Autodesk Inventor part; units mm, degrees
(part 8 of 8)
  spline S282 degree 3 poles (-4.5229, -9.4251) (-4.5278, -9.4188) (-4.5373, -9.4067) (-4.5516, -9.3896) (-4.5651, -9.3741) (-4.5784, -9.3606) (-4.5908, -9.3484) (-4.6028, -9.3379) (-4.6143, -9.3292) (-4.6288, -9.3198) (-4.647, -9.3105) (-4.6699, -9.3026) (-4.6937, -9.2979) (-4.71, -9.2972) (-4.7182, -9.2969) knots 0 0 0 0 0.098469 0.189629 0.274184 0.352183 0.423199 0.488551 0.548473 0.60144 0.701198 0.799592 0.898545 1 1 1 1
  spline S283 degree 3 poles (-4.7182, -9.2969) (-4.7286, -9.2973) (-4.7485, -9.2979) (-4.7768, -9.3052) (-4.8022, -9.3167) (-4.8241, -9.3328) (-4.8423, -9.3519) (-4.8555, -9.3738) (-4.8634, -9.398) (-4.8644, -9.4149) (-4.8649, -9.4235) knots 0 0 0 0 0.143073 0.275903 0.402371 0.528414 0.650356 0.765895 0.880774 1 1 1 1
  spline S284 degree 3 poles (-4.8649, -9.4235) (-4.8648, -9.4289) (-4.8645, -9.4396) (-4.8614, -9.4555) (-4.8574, -9.4713) (-4.851, -9.4869) (-4.8422, -9.5028) (-4.8306, -9.5191) (-4.816, -9.536) (-4.8049, -9.5469) (-4.799, -9.5527) knots 0 0 0 0 0.107285 0.214746 0.322939 0.434116 0.553412 0.686073 0.834256 1 1 1 1
  spline S285 degree 3 poles (-4.799, -9.5527) (-4.7968, -9.5547) (-4.7916, -9.5593) (-4.7821, -9.5669) (-4.7695, -9.5763) (-4.7542, -9.5879) (-4.736, -9.6013) (-4.7147, -9.6165) (-4.6906, -9.6338) (-4.6736, -9.6459) (-4.6646, -9.6523) knots 0 0 0 0 0.052594 0.124952 0.218094 0.333502 0.468789 0.624938 0.801683 1 1 1 1
  spline S286 degree 3 poles (-4.6646, -9.6523) (-4.6537, -9.6602) (-4.6327, -9.6755) (-4.6028, -9.6985) (-4.5757, -9.7209) (-4.5512, -9.7428) (-4.5293, -9.7638) (-4.51, -9.7842) (-4.4932, -9.8039) (-4.4752, -9.8293) (-4.4568, -9.8603) (-4.4409, -9.8984) (-4.4309, -9.9366) (-4.4296, -9.9623) (-4.429, -9.975) knots 0 0 0 0 0.096972 0.187773 0.272396 0.351321 0.424335 0.491909 0.554233 0.611268 0.716348 0.81454 0.908495 1 1 1 1
  line L313 (-4.1341, -10.22) -> (-4.2238, -10.22)
  line L314 (-4.2238, -10.22) -> (-4.2238, -9.22)
  line L315 (-4.2238, -9.22) -> (-4.0277, -9.22)
  spline S287 degree 3 poles (-4.0277, -9.22) (-4.0142, -9.22) (-3.9884, -9.22) (-3.9513, -9.2209) (-3.9177, -9.2221) (-3.8875, -9.2236) (-3.8607, -9.2255) (-3.8374, -9.2282) (-3.8174, -9.2309) (-3.8054, -9.2337) (-3.8, -9.235) knots 0 0 0 0 0.176956 0.339055 0.486318 0.618781 0.735619 0.838742 0.926457 1 1 1 1
  spline S288 degree 3 poles (-3.8, -9.235) (-3.7931, -9.2369) (-3.7794, -9.2407) (-3.7597, -9.2481) (-3.741, -9.257) (-3.7231, -9.2671) (-3.7064, -9.2789) (-3.6905, -9.2919) (-3.6757, -9.3064) (-3.6619, -9.3222) (-3.6493, -9.3391) (-3.6384, -9.3574) (-3.6292, -9.3766) (-3.6214, -9.3968) (-3.6158, -9.4182) (-3.6115, -9.4406) (-3.6089, -9.4641) (-3.6086, -9.4801) (-3.6085, -9.4882) knots 0 0 0 0 0.062481 0.12349 0.183411 0.243153 0.302127 0.36171 0.421842 0.482932 0.544552 0.605681 0.66768 0.729984 0.794551 0.860346 0.928907 1 1 1 1
  spline S289 degree 3 poles (-3.6085, -9.4882) (-3.6086, -9.4965) (-3.6088, -9.5125) (-3.6116, -9.5361) (-3.6155, -9.5586) (-3.6213, -9.58) (-3.629, -9.6001) (-3.638, -9.6194) (-3.6488, -9.6374) (-3.6613, -9.6543) (-3.6752, -9.67) (-3.6904, -9.6844) (-3.7069, -9.6974) (-3.7246, -9.7092) (-3.7437, -9.7193) (-3.764, -9.7284) (-3.7855, -9.736) (-3.8004, -9.74) (-3.808, -9.742) knots 0 0 0 0 0.070119 0.137192 0.202016 0.264631 0.326117 0.38601 0.445812 0.505298 0.564633 0.624283 0.683902 0.743953 0.805388 0.868388 0.933084 1 1 1 1
  spline S290 degree 3 poles (-3.808, -9.742) (-3.8142, -9.7434) (-3.828, -9.7463) (-3.8506, -9.7495) (-3.8769, -9.7523) (-3.9069, -9.7544) (-3.9406, -9.7562) (-3.9779, -9.7576) (-4.019, -9.7584) (-4.0476, -9.7584) (-4.0626, -9.7585) knots 0 0 0 0 0.075173 0.164746 0.268017 0.385912 0.517789 0.663691 0.824413 1 1 1 1
  line L316 (-4.0626, -9.7585) -> (-4.1341, -9.7585)
  line L317 (-4.1341, -9.7585) -> (-4.1341, -10.22)
  spline S291 degree 3 poles (-7.5315, -6.9138) (-7.5317, -6.9086) (-7.5319, -6.8982) (-7.5349, -6.883) (-7.5393, -6.8683) (-7.5455, -6.8541) (-7.5537, -6.8405) (-7.5635, -6.8275) (-7.5752, -6.815) (-7.5886, -6.8034) (-7.603, -6.7923) (-7.6188, -6.7829) (-7.6355, -6.7749) (-7.6531, -6.7682) (-7.6717, -6.7632) (-7.6912, -6.7596) (-7.7116, -6.7574) (-7.7256, -6.7571) (-7.7327, -6.7569) knots 0 0 0 0 0.055275 0.109966 0.163247 0.218076 0.273301 0.330909 0.390995 0.454176 0.518862 0.583311 0.648517 0.715031 0.782502 0.852323 0.924928 1 1 1 1
  spline S292 degree 3 poles (-7.7327, -6.7569) (-7.744, -6.7573) (-7.7663, -6.7581) (-7.7983, -6.7649) (-7.8282, -6.7757) (-7.8509, -6.7887) (-7.8678, -6.8015) (-7.8798, -6.8127) (-7.8916, -6.8251) (-7.9024, -6.8395) (-7.9133, -6.8549) (-7.9233, -6.8722) (-7.933, -6.8908) (-7.9388, -6.904) (-7.9418, -6.9108) knots 0 0 0 0 0.122712 0.239685 0.351816 0.463766 0.520818 0.579448 0.640604 0.705298 0.773634 0.844669 0.920057 1 1 1 1
  line L318 (-7.9418, -6.9108) -> (-8.0315, -6.9108)
  spline S293 degree 3 poles (-8.0315, -6.9108) (-8.0291, -6.9007) (-8.0244, -6.881) (-8.0144, -6.8529) (-8.0036, -6.8263) (-7.9907, -6.8017) (-7.9765, -6.7786) (-7.9603, -6.7576) (-7.9428, -6.738) (-7.9234, -6.7207) (-7.9031, -6.705) (-7.8815, -6.6916) (-7.8592, -6.6801) (-7.8359, -6.6706) (-7.8116, -6.6634) (-7.7865, -6.6582) (-7.7605, -6.6549) (-7.7428, -6.6545) (-7.7339, -6.6544) knots 0 0 0 0 0.072625 0.141977 0.208985 0.273957 0.336889 0.398745 0.460116 0.520825 0.580994 0.640152 0.698622 0.757271 0.816427 0.876254 0.937165 1 1 1 1
  spline S294 degree 3 poles (-7.7339, -6.6544) (-7.7208, -6.6548) (-7.695, -6.6555) (-7.6571, -6.6627) (-7.6205, -6.6739) (-7.5857, -6.6895) (-7.5533, -6.7087) (-7.5245, -6.7315) (-7.4997, -6.7576) (-7.4789, -6.7864) (-7.4626, -6.8171) (-7.4505, -6.8488) (-7.4432, -6.8813) (-7.4423, -6.9032) (-7.4418, -6.9142) knots 0 0 0 0 0.090254 0.17854 0.266093 0.354631 0.441886 0.525747 0.608114 0.690197 0.770821 0.848326 0.924012 1 1 1 1
  spline S295 degree 3 poles (-7.4418, -6.9142) (-7.4421, -6.9247) (-7.4428, -6.9454) (-7.4483, -6.9756) (-7.4576, -7.0041) (-7.4705, -7.031) (-7.4871, -7.056) (-7.5073, -7.0794) (-7.5312, -7.1011) (-7.5493, -7.1135) (-7.5586, -7.1199) knots 0 0 0 0 0.128068 0.250608 0.37063 0.490072 0.610375 0.734313 0.863217 1 1 1 1
  spline S296 degree 3 poles (-7.5586, -7.1199) (-7.5479, -7.125) (-7.5269, -7.1352) (-7.4981, -7.1552) (-7.4721, -7.1782) (-7.4575, -7.1962) (-7.4502, -7.2052) knots 0 0 0 0 0.25388 0.503009 0.750291 1 1 1 1
  spline S297 degree 3 poles (-7.4502, -7.2052) (-7.4454, -7.2118) (-7.4359, -7.2249) (-7.4241, -7.2459) (-7.4134, -7.2671) (-7.4051, -7.2892) (-7.3986, -7.3118) (-7.394, -7.335) (-7.3911, -7.3587) (-7.3907, -7.3748) (-7.3905, -7.3829) knots 0 0 0 0 0.128136 0.254173 0.378112 0.501712 0.623986 0.747096 0.872875 1 1 1 1
  spline S298 degree 3 poles (-7.3905, -7.3829) (-7.391, -7.3969) (-7.392, -7.4249) (-7.4012, -7.4661) (-7.4154, -7.5065) (-7.4355, -7.5451) (-7.46, -7.5812) (-7.4892, -7.6135) (-7.5227, -7.6413) (-7.5601, -7.6645) (-7.6006, -7.683) (-7.6439, -7.6959) (-7.6894, -7.7043) (-7.7206, -7.7052) (-7.7365, -7.7056) knots 0 0 0 0 0.079648 0.158922 0.239619 0.322609 0.406035 0.487602 0.569685 0.653036 0.737436 0.822478 0.909748 1 1 1 1
  spline S299 degree 3 poles (-7.7365, -7.7056) (-7.7472, -7.7054) (-7.7682, -7.7049) (-7.7991, -7.7016) (-7.8286, -7.6955) (-7.8568, -7.6873) (-7.8836, -7.6769) (-7.909, -7.6639) (-7.9331, -7.6487) (-7.9557, -7.631) (-7.9769, -7.6112) (-7.996, -7.589) (-8.0133, -7.5647) (-8.0284, -7.5381) (-8.042, -7.5095) (-8.0532, -7.4786) (-8.0631, -7.4456) (-8.0676, -7.4226) (-8.07, -7.4108) knots 0 0 0 0 0.065541 0.128963 0.190377 0.250092 0.308548 0.366398 0.424542 0.48317 0.542243 0.601739 0.662506 0.724856 0.789128 0.856346 0.926295 1 1 1 1
  line L319 (-8.07, -7.4108) -> (-7.9803, -7.4108)
  spline S300 degree 3 poles (-7.9803, -7.4108) (-7.9779, -7.4185) (-7.9734, -7.4334) (-7.9656, -7.455) (-7.9568, -7.4748) (-7.9473, -7.4929) (-7.9374, -7.5095) (-7.9263, -7.5242) (-7.9148, -7.5377) (-7.9062, -7.5453) (-7.9019, -7.549) knots 0 0 0 0 0.14977 0.291316 0.425966 0.55216 0.671527 0.786122 0.895325 1 1 1 1
  spline S301 degree 3 poles (-7.9019, -7.549) (-7.8963, -7.5533) (-7.8852, -7.5619) (-7.8669, -7.5729) (-7.8478, -7.5825) (-7.8273, -7.5897) (-7.8058, -7.5959) (-7.7831, -7.5999) (-7.7594, -7.6027) (-7.7432, -7.603) (-7.7349, -7.6031) knots 0 0 0 0 0.118271 0.236178 0.355663 0.475904 0.600127 0.728608 0.861313 1 1 1 1
  spline S302 degree 3 poles (-7.7349, -7.6031) (-7.7255, -7.6029) (-7.7072, -7.6026) (-7.6805, -7.5994) (-7.6551, -7.5948) (-7.6313, -7.5877) (-7.6087, -7.5789) (-7.5878, -7.5678) (-7.5681, -7.5549) (-7.55, -7.5401) (-7.5337, -7.524) (-7.5194, -7.5072) (-7.5072, -7.4896) (-7.4974, -7.4713) (-7.4897, -7.4524) (-7.4844, -7.4326) (-7.4807, -7.4123) (-7.4804, -7.3985) (-7.4803, -7.3915) knots 0 0 0 0 0.076072 0.148752 0.218403 0.28576 0.350598 0.414964 0.478069 0.541761 0.60435 0.664075 0.721464 0.777587 0.832644 0.887844 0.94346 1 1 1 1
  spline S303 degree 3 poles (-7.4803, -7.3915) (-7.4807, -7.3822) (-7.4816, -7.3636) (-7.4882, -7.3363) (-7.4992, -7.3099) (-7.5145, -7.285) (-7.5332, -7.262) (-7.555, -7.2414) (-7.5802, -7.2244) (-7.6033, -7.2126) (-7.6238, -7.2046) (-7.6414, -7.1993) (-7.661, -7.1948) (-7.6825, -7.1906) (-7.706, -7.187) (-7.7316, -7.184) (-7.7591, -7.1816) (-7.7781, -7.1805) (-7.7879, -7.18) knots 0 0 0 0 0.066909 0.133485 0.201035 0.271234 0.34288 0.413836 0.485977 0.56023 0.599884 0.644055 0.691892 0.744688 0.801492 0.862858 0.929328 1 1 1 1
  line L320 (-7.7879, -7.18) -> (-7.7879, -7.0774)
  spline S304 degree 3 poles (-7.7879, -7.0774) (-7.7756, -7.0772) (-7.7513, -7.0768) (-7.7159, -7.0718) (-7.6821, -7.065) (-7.6505, -7.0544) (-7.6218, -7.0422) (-7.5968, -7.0279) (-7.576, -7.0121) (-7.5595, -6.9944) (-7.5471, -6.9755) (-7.538, -6.9557) (-7.5326, -6.935) (-7.5319, -6.9209) (-7.5315, -6.9138) knots 0 0 0 0 0.110166 0.215787 0.318027 0.417574 0.51165 0.596162 0.672935 0.74367 0.810677 0.874059 0.936696 1 1 1 1
  spline S305 degree 3 poles (-6.6597, -6.9617) (-6.6601, -6.9721) (-6.6608, -6.9934) (-6.6655, -7.0258) (-6.6737, -7.0588) (-6.6829, -7.0867) (-6.6918, -7.1098) (-6.7001, -7.128) (-6.7094, -7.1471) (-6.7203, -7.1671) (-6.7319, -7.188) (-6.7451, -7.2097) (-6.7594, -7.2323) (-6.7697, -7.2475) (-6.7749, -7.2553) knots 0 0 0 0 0.09832 0.199417 0.305603 0.416162 0.474582 0.537006 0.603857 0.67409 0.749417 0.828253 0.912054 1 1 1 1
  line L321 (-6.7749, -7.2553) -> (-7.0828, -7.7056)
  line L322 (-7.0828, -7.7056) -> (-7.1545, -7.6558)
  line L323 (-7.1545, -7.6558) -> (-6.8765, -7.2493)
  spline S306 degree 3 poles (-6.8765, -7.2493) (-6.8942, -7.2515) (-6.9292, -7.2558) (-6.9643, -7.2565) (-6.9817, -7.2569) knots 0 0 0 0 0.507858 1 1 1 1
  spline S307 degree 3 poles (-6.9817, -7.2569) (-6.9922, -7.2567) (-7.0128, -7.2561) (-7.0431, -7.2519) (-7.0722, -7.2455) (-7.1, -7.2359) (-7.1267, -7.2239) (-7.1522, -7.2091) (-7.1764, -7.1917) (-7.1991, -7.1717) (-7.2198, -7.1498) (-7.2382, -7.1266) (-7.2535, -7.1019) (-7.2662, -7.0761) (-7.2758, -7.0489) (-7.2829, -7.0206) (-7.2872, -6.991) (-7.2877, -6.9709) (-7.2879, -6.9606) knots 0 0 0 0 0.066295 0.130131 0.192862 0.25436 0.31591 0.377338 0.440205 0.504175 0.568034 0.630228 0.690861 0.751422 0.811466 0.87275 0.935391 1 1 1 1
  spline S308 degree 3 poles (-7.2879, -6.9606) (-7.2875, -6.9467) (-7.2865, -6.9192) (-7.2787, -6.8791) (-7.2658, -6.8411) (-7.2478, -6.8055) (-7.2252, -6.7726) (-7.198, -6.743) (-7.1665, -6.7171) (-7.1312, -6.6948) (-7.0931, -6.6769) (-7.0532, -6.6637) (-7.0118, -6.6559) (-6.9838, -6.6549) (-6.9696, -6.6544) knots 0 0 0 0 0.085249 0.167327 0.248175 0.328829 0.409908 0.490584 0.572993 0.658265 0.744222 0.82906 0.913938 1 1 1 1
  spline S309 degree 3 poles (-6.9696, -6.6544) (-6.9558, -6.6549) (-6.9284, -6.6559) (-6.8882, -6.6635) (-6.8496, -6.6762) (-6.813, -6.6939) (-6.779, -6.716) (-6.7485, -6.7423) (-6.7221, -6.7728) (-6.6999, -6.8069) (-6.6821, -6.8435) (-6.6692, -6.8818) (-6.6612, -6.9213) (-6.6602, -6.9481) (-6.6597, -6.9617) knots 0 0 0 0 0.085532 0.169003 0.251943 0.335682 0.419409 0.501265 0.583703 0.668 0.751919 0.834598 0.916526 1 1 1 1
  spline S310 degree 3 poles (-7.5315, -1.8338) (-7.5317, -1.8286) (-7.5319, -1.8182) (-7.5349, -1.803) (-7.5393, -1.7883) (-7.5455, -1.7741) (-7.5537, -1.7605) (-7.5635, -1.7475) (-7.5752, -1.735) (-7.5886, -1.7234) (-7.603, -1.7123) (-7.6188, -1.7029) (-7.6355, -1.6949) (-7.6531, -1.6882) (-7.6717, -1.6832) (-7.6912, -1.6796) (-7.7116, -1.6774) (-7.7256, -1.6771) (-7.7327, -1.6769) knots 0 0 0 0 0.055275 0.109966 0.163247 0.218076 0.273301 0.330909 0.390995 0.454176 0.518862 0.583311 0.648517 0.715031 0.782502 0.852323 0.924928 1 1 1 1
  spline S311 degree 3 poles (-7.7327, -1.6769) (-7.744, -1.6773) (-7.7663, -1.6781) (-7.7983, -1.6849) (-7.8282, -1.6957) (-7.8509, -1.7087) (-7.8678, -1.7215) (-7.8798, -1.7327) (-7.8916, -1.7451) (-7.9024, -1.7595) (-7.9133, -1.7749) (-7.9233, -1.7922) (-7.933, -1.8108) (-7.9388, -1.824) (-7.9418, -1.8308) knots 0 0 0 0 0.122712 0.239685 0.351816 0.463766 0.520818 0.579448 0.640604 0.705298 0.773634 0.844669 0.920057 1 1 1 1
  line L324 (-7.9418, -1.8308) -> (-8.0315, -1.8308)
  spline S312 degree 3 poles (-8.0315, -1.8308) (-8.0291, -1.8207) (-8.0244, -1.801) (-8.0144, -1.7729) (-8.0036, -1.7463) (-7.9907, -1.7217) (-7.9765, -1.6986) (-7.9603, -1.6776) (-7.9428, -1.658) (-7.9234, -1.6407) (-7.9031, -1.625) (-7.8815, -1.6116) (-7.8592, -1.6001) (-7.8359, -1.5906) (-7.8116, -1.5834) (-7.7865, -1.5782) (-7.7605, -1.5749) (-7.7428, -1.5745) (-7.7339, -1.5744) knots 0 0 0 0 0.072625 0.141977 0.208985 0.273957 0.336889 0.398745 0.460116 0.520825 0.580994 0.640152 0.698622 0.757271 0.816427 0.876254 0.937165 1 1 1 1
  spline S313 degree 3 poles (-7.7339, -1.5744) (-7.7208, -1.5748) (-7.695, -1.5755) (-7.6571, -1.5827) (-7.6205, -1.5939) (-7.5857, -1.6095) (-7.5533, -1.6287) (-7.5245, -1.6515) (-7.4997, -1.6776) (-7.4789, -1.7064) (-7.4626, -1.7371) (-7.4505, -1.7688) (-7.4432, -1.8013) (-7.4423, -1.8232) (-7.4418, -1.8342) knots 0 0 0 0 0.090254 0.17854 0.266093 0.354631 0.441886 0.525747 0.608114 0.690197 0.770821 0.848326 0.924012 1 1 1 1
  spline S314 degree 3 poles (-7.4418, -1.8342) (-7.4421, -1.8447) (-7.4428, -1.8654) (-7.4483, -1.8956) (-7.4576, -1.9241) (-7.4705, -1.951) (-7.4871, -1.976) (-7.5073, -1.9994) (-7.5312, -2.0211) (-7.5493, -2.0335) (-7.5586, -2.0399) knots 0 0 0 0 0.128068 0.250608 0.37063 0.490072 0.610375 0.734313 0.863217 1 1 1 1
  spline S315 degree 3 poles (-7.5586, -2.0399) (-7.5479, -2.045) (-7.5269, -2.0552) (-7.4981, -2.0752) (-7.4721, -2.0982) (-7.4575, -2.1162) (-7.4502, -2.1252) knots 0 0 0 0 0.25388 0.503009 0.750291 1 1 1 1
  spline S316 degree 3 poles (-7.4502, -2.1252) (-7.4454, -2.1318) (-7.4359, -2.1449) (-7.4241, -2.1659) (-7.4134, -2.1871) (-7.4051, -2.2092) (-7.3986, -2.2318) (-7.394, -2.255) (-7.3911, -2.2787) (-7.3907, -2.2948) (-7.3905, -2.3029) knots 0 0 0 0 0.128136 0.254173 0.378112 0.501712 0.623986 0.747096 0.872875 1 1 1 1
  spline S317 degree 3 poles (-7.3905, -2.3029) (-7.391, -2.3169) (-7.392, -2.3449) (-7.4012, -2.3861) (-7.4154, -2.4265) (-7.4355, -2.4651) (-7.46, -2.5012) (-7.4892, -2.5335) (-7.5227, -2.5613) (-7.5601, -2.5845) (-7.6006, -2.603) (-7.6439, -2.6159) (-7.6894, -2.6243) (-7.7206, -2.6252) (-7.7365, -2.6256) knots 0 0 0 0 0.079648 0.158922 0.239619 0.322609 0.406035 0.487602 0.569685 0.653036 0.737436 0.822478 0.909748 1 1 1 1
  spline S318 degree 3 poles (-7.7365, -2.6256) (-7.7472, -2.6254) (-7.7682, -2.6249) (-7.7991, -2.6216) (-7.8286, -2.6155) (-7.8568, -2.6073) (-7.8836, -2.5969) (-7.909, -2.5839) (-7.9331, -2.5687) (-7.9557, -2.551) (-7.9769, -2.5312) (-7.996, -2.509) (-8.0133, -2.4847) (-8.0284, -2.4581) (-8.042, -2.4295) (-8.0532, -2.3986) (-8.0631, -2.3656) (-8.0676, -2.3426) (-8.07, -2.3308) knots 0 0 0 0 0.065541 0.128963 0.190377 0.250092 0.308548 0.366398 0.424542 0.48317 0.542243 0.601739 0.662506 0.724856 0.789128 0.856346 0.926295 1 1 1 1
  line L325 (-8.07, -2.3308) -> (-7.9803, -2.3308)
  spline S319 degree 3 poles (-7.9803, -2.3308) (-7.9779, -2.3385) (-7.9734, -2.3534) (-7.9656, -2.375) (-7.9568, -2.3948) (-7.9473, -2.4129) (-7.9374, -2.4295) (-7.9263, -2.4442) (-7.9148, -2.4577) (-7.9062, -2.4653) (-7.9019, -2.469) knots 0 0 0 0 0.14977 0.291316 0.425966 0.55216 0.671527 0.786122 0.895325 1 1 1 1
  spline S320 degree 3 poles (-7.9019, -2.469) (-7.8963, -2.4733) (-7.8852, -2.4819) (-7.8669, -2.4929) (-7.8478, -2.5025) (-7.8273, -2.5097) (-7.8058, -2.5159) (-7.7831, -2.5199) (-7.7594, -2.5227) (-7.7432, -2.523) (-7.7349, -2.5231) knots 0 0 0 0 0.118271 0.236178 0.355663 0.475904 0.600127 0.728608 0.861313 1 1 1 1
  spline S321 degree 3 poles (-7.7349, -2.5231) (-7.7255, -2.5229) (-7.7072, -2.5226) (-7.6805, -2.5194) (-7.6551, -2.5148) (-7.6313, -2.5077) (-7.6087, -2.4989) (-7.5878, -2.4878) (-7.5681, -2.4749) (-7.55, -2.4601) (-7.5337, -2.444) (-7.5194, -2.4272) (-7.5072, -2.4096) (-7.4974, -2.3913) (-7.4897, -2.3724) (-7.4844, -2.3526) (-7.4807, -2.3323) (-7.4804, -2.3185) (-7.4803, -2.3115) knots 0 0 0 0 0.076072 0.148752 0.218403 0.28576 0.350598 0.414964 0.478069 0.541761 0.60435 0.664075 0.721464 0.777587 0.832644 0.887844 0.94346 1 1 1 1
  spline S322 degree 3 poles (-7.4803, -2.3115) (-7.4807, -2.3022) (-7.4816, -2.2836) (-7.4882, -2.2563) (-7.4992, -2.2299) (-7.5145, -2.205) (-7.5332, -2.182) (-7.555, -2.1614) (-7.5802, -2.1444) (-7.6033, -2.1326) (-7.6238, -2.1246) (-7.6414, -2.1193) (-7.661, -2.1148) (-7.6825, -2.1106) (-7.706, -2.107) (-7.7316, -2.104) (-7.7591, -2.1016) (-7.7781, -2.1005) (-7.7879, -2.1) knots 0 0 0 0 0.066909 0.133485 0.201035 0.271234 0.34288 0.413836 0.485977 0.56023 0.599884 0.644055 0.691892 0.744688 0.801492 0.862858 0.929328 1 1 1 1
  line L326 (-7.7879, -2.1) -> (-7.7879, -1.9974)
  spline S323 degree 3 poles (-7.7879, -1.9974) (-7.7756, -1.9972) (-7.7513, -1.9968) (-7.7159, -1.9918) (-7.6821, -1.985) (-7.6505, -1.9744) (-7.6218, -1.9622) (-7.5968, -1.9479) (-7.576, -1.9321) (-7.5595, -1.9144) (-7.5471, -1.8955) (-7.538, -1.8757) (-7.5326, -1.855) (-7.5319, -1.8409) (-7.5315, -1.8338) knots 0 0 0 0 0.110166 0.215787 0.318027 0.417574 0.51165 0.596162 0.672935 0.74367 0.810677 0.874059 0.936696 1 1 1 1
  spline S324 degree 3 poles (-6.7623, -1.8338) (-6.7624, -1.8286) (-6.7627, -1.8182) (-6.7656, -1.803) (-6.7701, -1.7883) (-6.7762, -1.7741) (-6.7844, -1.7605) (-6.7943, -1.7475) (-6.806, -1.735) (-6.8194, -1.7234) (-6.8338, -1.7123) (-6.8496, -1.7029) (-6.8663, -1.6949) (-6.8839, -1.6882) (-6.9025, -1.6832) (-6.922, -1.6796) (-6.9424, -1.6774) (-6.9563, -1.6771) (-6.9634, -1.6769) knots 0 0 0 0 0.055275 0.109966 0.163247 0.218076 0.273301 0.330909 0.390995 0.454176 0.518862 0.583311 0.648517 0.715031 0.782502 0.852323 0.924928 1 1 1 1
  spline S325 degree 3 poles (-6.9634, -1.6769) (-6.9748, -1.6773) (-6.9971, -1.6781) (-7.0291, -1.6849) (-7.0589, -1.6957) (-7.0817, -1.7087) (-7.0985, -1.7215) (-7.1106, -1.7327) (-7.1224, -1.7451) (-7.1332, -1.7595) (-7.1441, -1.7749) (-7.1541, -1.7922) (-7.1637, -1.8108) (-7.1696, -1.824) (-7.1726, -1.8308) knots 0 0 0 0 0.122712 0.239685 0.351816 0.463766 0.520818 0.579448 0.640604 0.705298 0.773634 0.844669 0.920057 1 1 1 1
  line L327 (-7.1726, -1.8308) -> (-7.2623, -1.8308)
  spline S326 degree 3 poles (-7.2623, -1.8308) (-7.2599, -1.8207) (-7.2551, -1.801) (-7.2452, -1.7729) (-7.2344, -1.7463) (-7.2214, -1.7217) (-7.2073, -1.6986) (-7.1911, -1.6776) (-7.1736, -1.658) (-7.1542, -1.6407) (-7.1339, -1.625) (-7.1123, -1.6116) (-7.09, -1.6001) (-7.0667, -1.5906) (-7.0423, -1.5834) (-7.0172, -1.5782) (-6.9912, -1.5749) (-6.9736, -1.5745) (-6.9646, -1.5744) knots 0 0 0 0 0.072625 0.141977 0.208985 0.273957 0.336889 0.398745 0.460116 0.520825 0.580994 0.640152 0.698622 0.757271 0.816427 0.876254 0.937165 1 1 1 1
  spline S327 degree 3 poles (-6.9646, -1.5744) (-6.9516, -1.5748) (-6.9258, -1.5755) (-6.8878, -1.5827) (-6.8512, -1.5939) (-6.8164, -1.6095) (-6.7841, -1.6287) (-6.7553, -1.6515) (-6.7305, -1.6776) (-6.7096, -1.7064) (-6.6933, -1.7371) (-6.6813, -1.7688) (-6.674, -1.8013) (-6.673, -1.8232) (-6.6726, -1.8342) knots 0 0 0 0 0.090254 0.17854 0.266093 0.354631 0.441886 0.525747 0.608114 0.690197 0.770821 0.848326 0.924012 1 1 1 1
  spline S328 degree 3 poles (-6.6726, -1.8342) (-6.6729, -1.8447) (-6.6735, -1.8654) (-6.6791, -1.8956) (-6.6884, -1.9241) (-6.7012, -1.951) (-6.7179, -1.976) (-6.7381, -1.9994) (-6.762, -2.0211) (-6.78, -2.0335) (-6.7894, -2.0399) knots 0 0 0 0 0.128068 0.250608 0.37063 0.490072 0.610375 0.734313 0.863217 1 1 1 1
  spline S329 degree 3 poles (-6.7894, -2.0399) (-6.7787, -2.045) (-6.7576, -2.0552) (-6.7289, -2.0752) (-6.7028, -2.0982) (-6.6883, -2.1162) (-6.681, -2.1252) knots 0 0 0 0 0.25388 0.503009 0.750291 1 1 1 1
  spline S330 degree 3 poles (-6.681, -2.1252) (-6.6762, -2.1318) (-6.6666, -2.1449) (-6.6548, -2.1659) (-6.6442, -2.1871) (-6.6358, -2.2092) (-6.6294, -2.2318) (-6.6248, -2.255) (-6.6219, -2.2787) (-6.6215, -2.2948) (-6.6213, -2.3029) knots 0 0 0 0 0.128136 0.254173 0.378112 0.501712 0.623986 0.747096 0.872875 1 1 1 1
  spline S331 degree 3 poles (-6.6213, -2.3029) (-6.6218, -2.3169) (-6.6228, -2.3449) (-6.632, -2.3861) (-6.6461, -2.4265) (-6.6663, -2.4651) (-6.6908, -2.5012) (-6.72, -2.5335) (-6.7535, -2.5613) (-6.7909, -2.5845) (-6.8314, -2.603) (-6.8747, -2.6159) (-6.9202, -2.6243) (-6.9514, -2.6252) (-6.9672, -2.6256) knots 0 0 0 0 0.079648 0.158922 0.239619 0.322609 0.406035 0.487602 0.569685 0.653036 0.737436 0.822478 0.909748 1 1 1 1
  spline S332 degree 3 poles (-6.9672, -2.6256) (-6.9779, -2.6254) (-6.999, -2.6249) (-7.0299, -2.6216) (-7.0594, -2.6155) (-7.0876, -2.6073) (-7.1144, -2.5969) (-7.1398, -2.5839) (-7.1639, -2.5687) (-7.1865, -2.551) (-7.2076, -2.5312) (-7.2267, -2.509) (-7.2441, -2.4847) (-7.2592, -2.4581) (-7.2728, -2.4295) (-7.284, -2.3986) (-7.2938, -2.3656) (-7.2984, -2.3426) (-7.3008, -2.3308) knots 0 0 0 0 0.065541 0.128963 0.190377 0.250092 0.308548 0.366398 0.424542 0.48317 0.542243 0.601739 0.662506 0.724856 0.789128 0.856346 0.926295 1 1 1 1
  line L328 (-7.3008, -2.3308) -> (-7.211, -2.3308)
  spline S333 degree 3 poles (-7.211, -2.3308) (-7.2087, -2.3385) (-7.2041, -2.3534) (-7.1964, -2.375) (-7.1876, -2.3948) (-7.1781, -2.4129) (-7.1682, -2.4295) (-7.1571, -2.4442) (-7.1456, -2.4577) (-7.1369, -2.4653) (-7.1327, -2.469) knots 0 0 0 0 0.14977 0.291316 0.425966 0.55216 0.671527 0.786122 0.895325 1 1 1 1
  spline S334 degree 3 poles (-7.1327, -2.469) (-7.1271, -2.4733) (-7.1159, -2.4819) (-7.0977, -2.4929) (-7.0785, -2.5025) (-7.058, -2.5097) (-7.0366, -2.5159) (-7.0139, -2.5199) (-6.9901, -2.5227) (-6.9739, -2.523) (-6.9656, -2.5231) knots 0 0 0 0 0.118271 0.236178 0.355663 0.475904 0.600127 0.728608 0.861313 1 1 1 1
  spline S335 degree 3 poles (-6.9656, -2.5231) (-6.9563, -2.5229) (-6.938, -2.5226) (-6.9113, -2.5194) (-6.8859, -2.5148) (-6.8621, -2.5077) (-6.8395, -2.4989) (-6.8185, -2.4878) (-6.7989, -2.4749) (-6.7808, -2.4601) (-6.7645, -2.444) (-6.7502, -2.4272) (-6.738, -2.4096) (-6.7282, -2.3913) (-6.7204, -2.3724) (-6.7151, -2.3526) (-6.7115, -2.3323) (-6.7112, -2.3185) (-6.711, -2.3115) knots 0 0 0 0 0.076072 0.148752 0.218403 0.28576 0.350598 0.414964 0.478069 0.541761 0.60435 0.664075 0.721464 0.777587 0.832644 0.887844 0.94346 1 1 1 1
  spline S336 degree 3 poles (-6.711, -2.3115) (-6.7115, -2.3022) (-6.7123, -2.2836) (-6.719, -2.2563) (-6.7299, -2.2299) (-6.7453, -2.205) (-6.764, -2.182) (-6.7858, -2.1614) (-6.8109, -2.1444) (-6.8341, -2.1326) (-6.8546, -2.1246) (-6.8721, -2.1193) (-6.8918, -2.1148) (-6.9133, -2.1106) (-6.9368, -2.107) (-6.9623, -2.104) (-6.9898, -2.1016) (-7.0089, -2.1005) (-7.0187, -2.1) knots 0 0 0 0 0.066909 0.133485 0.201035 0.271234 0.34288 0.413836 0.485977 0.56023 0.599884 0.644055 0.691892 0.744688 0.801492 0.862858 0.929328 1 1 1 1
  line L329 (-7.0187, -2.1) -> (-7.0187, -1.9974)
  spline S337 degree 3 poles (-7.0187, -1.9974) (-7.0063, -1.9972) (-6.9821, -1.9968) (-6.9467, -1.9918) (-6.9129, -1.985) (-6.8813, -1.9744) (-6.8526, -1.9622) (-6.8276, -1.9479) (-6.8068, -1.9321) (-6.7903, -1.9144) (-6.7779, -1.8955) (-6.7688, -1.8757) (-6.7634, -1.855) (-6.7627, -1.8409) (-6.7623, -1.8338) knots 0 0 0 0 0.110166 0.215787 0.318027 0.417574 0.51165 0.596162 0.672935 0.74367 0.810677 0.874059 0.936696 1 1 1 1
  spline S338 degree 3 poles (-7.5315, 0.7062) (-7.5317, 0.7114) (-7.5319, 0.7218) (-7.5349, 0.737) (-7.5393, 0.7517) (-7.5455, 0.7659) (-7.5537, 0.7795) (-7.5635, 0.7925) (-7.5752, 0.805) (-7.5886, 0.8166) (-7.603, 0.8277) (-7.6188, 0.8371) (-7.6355, 0.8451) (-7.6531, 0.8518) (-7.6717, 0.8568) (-7.6912, 0.8604) (-7.7116, 0.8626) (-7.7256, 0.8629) (-7.7327, 0.8631) knots 0 0 0 0 0.055275 0.109966 0.163247 0.218076 0.273301 0.330909 0.390995 0.454176 0.518862 0.583311 0.648517 0.715031 0.782502 0.852323 0.924928 1 1 1 1
  spline S339 degree 3 poles (-7.7327, 0.8631) (-7.744, 0.8627) (-7.7663, 0.8619) (-7.7983, 0.8551) (-7.8282, 0.8443) (-7.8509, 0.8313) (-7.8678, 0.8185) (-7.8798, 0.8073) (-7.8916, 0.7949) (-7.9024, 0.7805) (-7.9133, 0.7651) (-7.9233, 0.7478) (-7.933, 0.7292) (-7.9388, 0.716) (-7.9418, 0.7092) knots 0 0 0 0 0.122712 0.239685 0.351816 0.463766 0.520818 0.579448 0.640604 0.705298 0.773634 0.844669 0.920057 1 1 1 1
  line L330 (-7.9418, 0.7092) -> (-8.0315, 0.7092)
  spline S340 degree 3 poles (-8.0315, 0.7092) (-8.0291, 0.7193) (-8.0244, 0.739) (-8.0144, 0.7671) (-8.0036, 0.7937) (-7.9907, 0.8183) (-7.9765, 0.8414) (-7.9603, 0.8624) (-7.9428, 0.882) (-7.9234, 0.8993) (-7.9031, 0.915) (-7.8815, 0.9284) (-7.8592, 0.9399) (-7.8359, 0.9494) (-7.8116, 0.9566) (-7.7865, 0.9618) (-7.7605, 0.9651) (-7.7428, 0.9655) (-7.7339, 0.9656) knots 0 0 0 0 0.072625 0.141977 0.208985 0.273957 0.336889 0.398745 0.460116 0.520825 0.580994 0.640152 0.698622 0.757271 0.816427 0.876254 0.937165 1 1 1 1
  spline S341 degree 3 poles (-7.7339, 0.9656) (-7.7208, 0.9652) (-7.695, 0.9645) (-7.6571, 0.9573) (-7.6205, 0.9461) (-7.5857, 0.9305) (-7.5533, 0.9113) (-7.5245, 0.8885) (-7.4997, 0.8624) (-7.4789, 0.8336) (-7.4626, 0.8029) (-7.4505, 0.7712) (-7.4432, 0.7387) (-7.4423, 0.7168) (-7.4418, 0.7058) knots 0 0 0 0 0.090254 0.17854 0.266093 0.354631 0.441886 0.525747 0.608114 0.690197 0.770821 0.848326 0.924012 1 1 1 1
  spline S342 degree 3 poles (-7.4418, 0.7058) (-7.4421, 0.6953) (-7.4428, 0.6746) (-7.4483, 0.6444) (-7.4576, 0.6159) (-7.4705, 0.589) (-7.4871, 0.564) (-7.5073, 0.5406) (-7.5312, 0.5189) (-7.5493, 0.5065) (-7.5586, 0.5001) knots 0 0 0 0 0.128068 0.250608 0.37063 0.490072 0.610375 0.734313 0.863217 1 1 1 1
  spline S343 degree 3 poles (-7.5586, 0.5001) (-7.5479, 0.495) (-7.5269, 0.4848) (-7.4981, 0.4648) (-7.4721, 0.4418) (-7.4575, 0.4238) (-7.4502, 0.4148) knots 0 0 0 0 0.25388 0.503009 0.750291 1 1 1 1
  spline S344 degree 3 poles (-7.4502, 0.4148) (-7.4454, 0.4082) (-7.4359, 0.3951) (-7.4241, 0.3741) (-7.4134, 0.3529) (-7.4051, 0.3308) (-7.3986, 0.3082) (-7.394, 0.285) (-7.3911, 0.2613) (-7.3907, 0.2452) (-7.3905, 0.2371) knots 0 0 0 0 0.128136 0.254173 0.378112 0.501712 0.623986 0.747096 0.872875 1 1 1 1
  spline S345 degree 3 poles (-7.3905, 0.2371) (-7.391, 0.2231) (-7.392, 0.1951) (-7.4012, 0.1539) (-7.4154, 0.1135) (-7.4355, 0.0749) (-7.46, 0.0388) (-7.4892, 0.0065) (-7.5227, -0.0213) (-7.5601, -0.0445) (-7.6006, -0.063) (-7.6439, -0.0759) (-7.6894, -0.0843) (-7.7206, -0.0852) (-7.7365, -0.0856) knots 0 0 0 0 0.079648 0.158922 0.239619 0.322609 0.406035 0.487602 0.569685 0.653036 0.737436 0.822478 0.909748 1 1 1 1
  spline S346 degree 3 poles (-7.7365, -0.0856) (-7.7472, -0.0854) (-7.7682, -0.0849) (-7.7991, -0.0816) (-7.8286, -0.0755) (-7.8568, -0.0673) (-7.8836, -0.0569) (-7.909, -0.0439) (-7.9331, -0.0287) (-7.9557, -0.011) (-7.9769, 0.0088) (-7.996, 0.031) (-8.0133, 0.0553) (-8.0284, 0.0819) (-8.042, 0.1105) (-8.0532, 0.1414) (-8.0631, 0.1744) (-8.0676, 0.1974) (-8.07, 0.2092) knots 0 0 0 0 0.065541 0.128963 0.190377 0.250092 0.308548 0.366398 0.424542 0.48317 0.542243 0.601739 0.662506 0.724856 0.789128 0.856346 0.926295 1 1 1 1
  line L331 (-8.07, 0.2092) -> (-7.9803, 0.2092)
  spline S347 degree 3 poles (-7.9803, 0.2092) (-7.9779, 0.2015) (-7.9734, 0.1866) (-7.9656, 0.165) (-7.9568, 0.1452) (-7.9473, 0.1271) (-7.9374, 0.1105) (-7.9263, 0.0958) (-7.9148, 0.0823) (-7.9062, 0.0747) (-7.9019, 0.071) knots 0 0 0 0 0.14977 0.291316 0.425966 0.55216 0.671527 0.786122 0.895325 1 1 1 1
  spline S348 degree 3 poles (-7.9019, 0.071) (-7.8963, 0.0667) (-7.8852, 0.0581) (-7.8669, 0.0471) (-7.8478, 0.0375) (-7.8273, 0.0303) (-7.8058, 0.0241) (-7.7831, 0.0201) (-7.7594, 0.0173) (-7.7432, 0.017) (-7.7349, 0.0169) knots 0 0 0 0 0.118271 0.236178 0.355663 0.475904 0.600127 0.728608 0.861313 1 1 1 1
  spline S349 degree 3 poles (-7.7349, 0.0169) (-7.7255, 0.0171) (-7.7072, 0.0174) (-7.6805, 0.0206) (-7.6551, 0.0252) (-7.6313, 0.0323) (-7.6087, 0.0411) (-7.5878, 0.0522) (-7.5681, 0.0651) (-7.55, 0.0799) (-7.5337, 0.096) (-7.5194, 0.1128) (-7.5072, 0.1304) (-7.4974, 0.1487) (-7.4897, 0.1676) (-7.4844, 0.1874) (-7.4807, 0.2077) (-7.4804, 0.2215) (-7.4803, 0.2285) knots 0 0 0 0 0.076072 0.148752 0.218403 0.28576 0.350598 0.414964 0.478069 0.541761 0.60435 0.664075 0.721464 0.777587 0.832644 0.887844 0.94346 1 1 1 1
  spline S350 degree 3 poles (-7.4803, 0.2285) (-7.4807, 0.2378) (-7.4816, 0.2564) (-7.4882, 0.2837) (-7.4992, 0.3101) (-7.5145, 0.335) (-7.5332, 0.358) (-7.555, 0.3786) (-7.5802, 0.3956) (-7.6033, 0.4074) (-7.6238, 0.4154) (-7.6414, 0.4207) (-7.661, 0.4252) (-7.6825, 0.4294) (-7.706, 0.433) (-7.7316, 0.436) (-7.7591, 0.4384) (-7.7781, 0.4395) (-7.7879, 0.44) knots 0 0 0 0 0.066909 0.133485 0.201035 0.271234 0.34288 0.413836 0.485977 0.56023 0.599884 0.644055 0.691892 0.744688 0.801492 0.862858 0.929328 1 1 1 1
  line L332 (-7.7879, 0.44) -> (-7.7879, 0.5426)
  spline S351 degree 3 poles (-7.7879, 0.5426) (-7.7756, 0.5428) (-7.7513, 0.5432) (-7.7159, 0.5482) (-7.6821, 0.555) (-7.6505, 0.5656) (-7.6218, 0.5778) (-7.5968, 0.5921) (-7.576, 0.6079) (-7.5595, 0.6256) (-7.5471, 0.6445) (-7.538, 0.6643) (-7.5326, 0.685) (-7.5319, 0.6991) (-7.5315, 0.7062) knots 0 0 0 0 0.110166 0.215787 0.318027 0.417574 0.51165 0.596162 0.672935 0.74367 0.810677 0.874059 0.936696 1 1 1 1
  line L333 (-6.8264, 0.1708) -> (-7.3008, 0.1708)
  line L334 (-7.3008, 0.1708) -> (-6.7549, 0.9656)
  line L335 (-6.7549, 0.9656) -> (-6.7367, 0.9656)
  line L336 (-6.7367, 0.9656) -> (-6.7367, 0.2733)
  line L337 (-6.7367, 0.2733) -> (-6.6213, 0.2733)
  line L338 (-6.6213, 0.2733) -> (-6.6213, 0.1708)
  line L339 (-6.6213, 0.1708) -> (-6.7367, 0.1708)
  line L340 (-6.7367, 0.1708) -> (-6.7367, -0.06)
  line L341 (-6.7367, -0.06) -> (-6.8264, -0.06)
  line L342 (-6.8264, -0.06) -> (-6.8264, 0.1708)
  line L343 (-3.1854, 2.98) -> (-3.0828, 3.48)
  line L344 (-3.0828, 3.48) -> (-2.6726, 3.48)
  line L345 (-2.6726, 3.48) -> (-2.6726, 3.3774)
  line L346 (-2.6726, 3.3774) -> (-3.0127, 3.3774)
  line L347 (-3.0127, 3.3774) -> (-3.0666, 3.1144)
  spline S352 degree 3 poles (-3.0666, 3.1144) (-3.056, 3.1173) (-3.0355, 3.123) (-3.0052, 3.1293) (-2.9765, 3.1331) (-2.9578, 3.1336) (-2.9488, 3.1338) knots 0 0 0 0 0.275068 0.532901 0.773973 1 1 1 1
  spline S353 degree 3 poles (-2.9488, 3.1338) (-2.9376, 3.1336) (-2.9157, 3.1331) (-2.8836, 3.1286) (-2.8529, 3.1214) (-2.8237, 3.1113) (-2.7961, 3.0985) (-2.7701, 3.0825) (-2.7455, 3.0638) (-2.7227, 3.0422) (-2.7019, 3.0185) (-2.6837, 2.9931) (-2.6682, 2.9661) (-2.6558, 2.9373) (-2.6459, 2.907) (-2.6393, 2.8749) (-2.6348, 2.8414) (-2.6344, 2.8184) (-2.6341, 2.8067) knots 0 0 0 0 0.065808 0.129394 0.190894 0.251281 0.310815 0.370371 0.430768 0.492881 0.555104 0.616067 0.677256 0.73826 0.800762 0.864778 0.931045 1 1 1 1
  spline S354 degree 3 poles (-2.6341, 2.8067) (-2.6343, 2.7986) (-2.6347, 2.7824) (-2.6366, 2.7583) (-2.6403, 2.7348) (-2.6452, 2.7118) (-2.6517, 2.6893) (-2.6595, 2.6673) (-2.669, 2.6459) (-2.6795, 2.625) (-2.6913, 2.6049) (-2.7044, 2.5862) (-2.7182, 2.5684) (-2.733, 2.5519) (-2.7491, 2.5367) (-2.7662, 2.5227) (-2.7841, 2.5097) (-2.8031, 2.4982) (-2.8229, 2.4877) (-2.8436, 2.479) (-2.8649, 2.4713) (-2.887, 2.4651) (-2.9099, 2.4603) (-2.9336, 2.457) (-2.958, 2.4546) (-2.9745, 2.4544) (-2.9829, 2.4544) knots 0 0 0 0 0.044014 0.087434 0.130118 0.172554 0.214555 0.256298 0.298438 0.340849 0.382715 0.423924 0.464246 0.504074 0.543862 0.583567 0.623094 0.663229 0.703551 0.743938 0.784541 0.82575 0.867757 0.910745 0.954914 1 1 1 1
  spline S355 degree 3 poles (-2.9829, 2.4544) (-2.9928, 2.4546) (-3.0124, 2.4549) (-3.0411, 2.459) (-3.0688, 2.4648) (-3.0951, 2.4736) (-3.1204, 2.4845) (-3.1442, 2.4984) (-3.1672, 2.5141) (-3.1885, 2.5327) (-3.2083, 2.5529) (-3.226, 2.5749) (-3.2417, 2.5983) (-3.2553, 2.6231) (-3.2668, 2.6493) (-3.2759, 2.6771) (-3.2833, 2.7062) (-3.2864, 2.7262) (-3.2879, 2.7364) knots 0 0 0 0 0.065421 0.128708 0.190236 0.250724 0.310637 0.370766 0.431615 0.493523 0.555883 0.617342 0.678668 0.740711 0.802985 0.866803 0.932347 1 1 1 1
  line L348 (-3.2879, 2.7364) -> (-3.1982, 2.7364)
  spline S356 degree 3 poles (-3.1982, 2.7364) (-3.196, 2.7269) (-3.1918, 2.7085) (-3.1824, 2.6828) (-3.171, 2.6598) (-3.1575, 2.6394) (-3.1413, 2.6216) (-3.1229, 2.6057) (-3.1022, 2.5913) (-3.0793, 2.5794) (-3.055, 2.5692) (-3.0297, 2.5624) (-3.0039, 2.5576) (-2.9864, 2.5572) (-2.9777, 2.5569) knots 0 0 0 0 0.094687 0.181994 0.264377 0.34218 0.418618 0.496509 0.577369 0.661511 0.746733 0.831258 0.915206 1 1 1 1
  spline S357 degree 3 poles (-2.9777, 2.5569) (-2.9691, 2.5572) (-2.9522, 2.5576) (-2.9274, 2.5612) (-2.9035, 2.5666) (-2.8806, 2.5748) (-2.8585, 2.5848) (-2.8376, 2.5976) (-2.8173, 2.6123) (-2.7983, 2.6291) (-2.7809, 2.6477) (-2.7656, 2.6675) (-2.7528, 2.6887) (-2.742, 2.7108) (-2.7338, 2.7342) (-2.728, 2.7586) (-2.7246, 2.7842) (-2.7241, 2.8016) (-2.7238, 2.8105) knots 0 0 0 0 0.064207 0.126425 0.18768 0.248216 0.308305 0.369661 0.431699 0.495947 0.559758 0.622295 0.683911 0.745092 0.80674 0.869087 0.93329 1 1 1 1
  spline S358 degree 3 poles (-2.7238, 2.8105) (-2.724, 2.8186) (-2.7244, 2.8343) (-2.7274, 2.8572) (-2.7326, 2.879) (-2.7399, 2.8996) (-2.7491, 2.9191) (-2.7604, 2.9375) (-2.7739, 2.9545) (-2.7894, 2.9703) (-2.8063, 2.9848) (-2.825, 2.9972) (-2.8451, 3.0076) (-2.8663, 3.0166) (-2.8891, 3.023) (-2.9132, 3.0279) (-2.9387, 3.0307) (-2.9561, 3.0311) (-2.965, 3.0313) knots 0 0 0 0 0.065351 0.127916 0.18836 0.247216 0.30563 0.36377 0.422661 0.482687 0.5433 0.604118 0.664965 0.727413 0.791468 0.858055 0.927037 1 1 1 1
  spline S359 degree 3 poles (-2.965, 3.0313) (-2.9728, 3.0311) (-2.9888, 3.0308) (-3.0133, 3.0283) (-3.0391, 3.0242) (-3.0661, 3.0186) (-3.0943, 3.0113) (-3.1236, 3.0025) (-3.1542, 2.992) (-3.1748, 2.9841) (-3.1854, 2.98) knots 0 0 0 0 0.102203 0.211023 0.3251 0.446502 0.573788 0.708901 0.850358 1 1 1 1
  line L349 (-7.7623, 3.3774) -> (-7.9162, 3.3774)
  line L350 (-7.9162, 3.3774) -> (-7.8575, 3.48)
  line L351 (-7.8575, 3.48) -> (-7.6726, 3.48)
  line L352 (-7.6726, 3.48) -> (-7.6726, 2.48)
  line L353 (-7.6726, 2.48) -> (-7.7623, 2.48)
  line L354 (-7.7623, 2.48) -> (-7.7623, 3.3774)
  line L355 (-6.8264, 2.7108) -> (-7.3008, 2.7108)
  line L356 (-7.3008, 2.7108) -> (-6.7549, 3.5056)
  line L357 (-6.7549, 3.5056) -> (-6.7367, 3.5056)
  line L358 (-6.7367, 3.5056) -> (-6.7367, 2.8133)
  line L359 (-6.7367, 2.8133) -> (-6.6213, 2.8133)
  line L360 (-6.6213, 2.8133) -> (-6.6213, 2.7108)
  line L361 (-6.6213, 2.7108) -> (-6.7367, 2.7108)
  line L362 (-6.7367, 2.7108) -> (-6.7367, 2.48)
  line L363 (-6.7367, 2.48) -> (-6.8264, 2.48)
  line L364 (-6.8264, 2.48) -> (-6.8264, 2.7108)
  line L365 (-12.73, 5.52) -> (-12.73, -12.26)
  arc A17 (-10.13, 5.52) -> (-12.73, 5.52) centre (-11.43, 5.52) ccw
  line L366 (-10.13, -12.26) -> (-10.13, 5.52)
  arc A18 (-12.73, -12.26) -> (-10.13, -12.26) centre (-11.43, -12.26) ccw
  circle A19 centre (-11.43, 10.6) radius 0.75
  circle A20 centre (11.43, 10.6) radius 0.75
  circle A21 centre (-13.97, -9.72) radius 0.75
  circle A22 centre (13.97, -12.26) radius 0.75
  circle A23 centre (-13.97, -7.18) radius 0.75
  circle A24 centre (-13.97, -4.64) radius 0.75
  circle A25 centre (-13.97, 2.98) radius 0.75
  circle A26 centre (-12.2, 16.55) radius 0.65
  circle A27 centre (-13.97, 10.6) radius 0.75
  circle A28 centre (13.97, -2.1) radius 0.75
  circle A29 centre (13.97, -7.18) radius 0.75
  circle A30 centre (13.97, 5.52) radius 0.75
  circle A31 centre (13.97, 0.44) radius 0.75
  circle A32 centre (2.425, 13.35) radius 0.4
  circle A33 centre (-2.425, 13.35) radius 0.4
  line L367 (3, 16.65) -> (3, 15.95)
  arc A34 (3.7, 16.65) -> (3, 16.65) centre (3.35, 16.65) ccw
  line L368 (3.7, 15.95) -> (3.7, 16.65)
  arc A35 (3, 15.95) -> (3.7, 15.95) centre (3.35, 15.95) ccw
  line L369 (-3.7, 16.65) -> (-3.7, 15.95)
  arc A36 (-3, 16.65) -> (-3.7, 16.65) centre (-3.35, 16.65) ccw
  line L370 (-3, 15.95) -> (-3, 16.65)
  arc A37 (-3.7, 15.95) -> (-3, 15.95) centre (-3.35, 15.95) ccw
  line L371 (-4.1, 20) -> (-4.1, 18.85)
  arc A38 (-4.1, 18.85) -> (-3.9, 18.65) centre (-3.9, 18.85) ccw
  line L372 (-3.9, 18.65) -> (3.9, 18.65)
  arc A39 (3.9, 18.65) -> (4.1, 18.85) centre (3.9, 18.85) ccw
  line L373 (4.1, 18.85) -> (4.1, 20)
  line L374 (4.1, 20) -> (16, 20)
  line L375 (16, 20) -> (16, -17.2071)
  line L376 (16, -17.2071) -> (13.2071, -20)
  line L377 (13.2071, -20) -> (-13.2071, -20)
  line L378 (-13.2071, -20) -> (-16, -17.2071)
  line L379 (-16, -17.2071) -> (-16, 13.3)
  line L380 (-16, 13.3) -> (-14.1, 13.3)
  arc A40 (-14.1, 13.3) -> (-13.4, 14) centre (-14.1, 14) ccw
  line L381 (-13.4, 14) -> (-13.4, 20)
  line L382 (-13.4, 20) -> (-4.1, 20)
  line L383 (-13.4, 20) -> (-16, 20)
  line L384 (-16, 20) -> (-16, 13.3)
  line L385 (-16, 13.3) -> (-13.4, 13.3)
  line L386 (-13.4, 13.3) -> (-13.4, 20)
  point P0 (0, 0)
  dimension "d9" = 0.5
  constraints: 32 end point, 6 point on circle, 3 centre point, 2 parallel, 1 horizontal, 1 perpendicular, 14 other
  measures "d9" distance between parallel lines of L3 L382
extrude "Extrusion5" cut sketch "Skizze5" against normal blind 4.3 contours L0 L11 L10 L9 L8 L7 L6 L5 A2 L4 L3 L2 A1 L1 A0 | A3 | A4 | A5 | A6 | A7 | A8 | A9 | A10 | L13 L14 L15 L12 | A11 | A12 | A13 | A14 | A15 L17 A16 L16 | S0 L18 L19 L20 S1 S2 S3 S4 | L21 L22 L23 L24 L25 L26 L27 | S5 S6 L28 S7 S8 S9 S10 S11 S12 S13 L29 S14 S15 S16 S17 L30 S18 | S19 S20 S21 S22 | S23 S24 L31 S25 S26 S27 S28 S29 S30 S31 L32 S32 S33 S34 S35 L33 S36 | S37 S38 S39 S40 | S41 S42 L34 S43 S44 S45 S46 S47 S48 S49 L35 S50 S51 S52 S53 L36 S54 | S55 S56 L37 S57 S58 S59 L38 L39 L40 L41 L42 S60 | S61 L43 L44 L45 S62 S63 S64 S65 | L46 L47 L48 L49 L50 L51 | L52 L53 L54 L55 L56 S66 S67 S68 S69 L57 S70 S71 S72 S73 | S74 S75 L58 S76 S77 S78 S79 S80 S81 S82 L59 S83 S84 S85 S86 L60 S87 | S88 S89 S90 S91 S92 S93 S94 S95 S96 | L61 L62 L63 L64 L65 L66 | S97 L67 L68 L69 S98 S99 S100 S101 | S102 S103 L70 S104 S105 S106 L71 L72 L73 L74 L75 S107 | L76 L77 L78 L79 L80 L81 L82 | S108 L83 L84 L85 S109 S110 | L86 L87 L88 L89 L90 L91 L92 L93 L94 L95 | S111 S112 L96 S113 S114 S115 S116 L97 L98 L99 S117 S118 S119 | L100 L101 L102 L103 L104 L105 L106 L107 | S120 S121 L108 S122 S123 S124 S125 S126 S127 S128 S129 L109 S130 S131 S132 S133 S134 | S135 S136 S137 S138 | L110 L111 L112 L113 L114 L115 L116 | S139 L117 L118 L119 S140 S141 | S142 S143 S144 S145 | L120 L121 L122 L123 L124 L125 | S146 S147 S148 S149 | L126 L127 L128 S150 S151 S152 L129 L130 L131 L132 L133 | L134 L135 L136 L137 L138 L139 L140 L141 L142 L143 L144 L145 | S153 S154 L146 S155 S156 S157 L147 L148 L149 L150 L151 S158 | L152 L153 L154 L155 L156 L157 | S159 S160 L158 S161 S162 S163 S164 L159 L160 L161 S165 S166 S167 | L162 L163 L164 L165 L166 L167 L168 L169 L170 L171 | L172 L173 L174 L175 L176 L177 L178 L179 L180 L181 L182 L183 | L184 L185 L186 L187 L188 L189 L190 L191 | S168 L192 L193 L194 S169 S170 | L195 L196 L197 L198 L199 S171 S172 S173 S174 L200 S175 S176 S177 S178 | S179 S180 L201 S181 S182 S183 L202 L203 L204 L205 L206 S184 | S185 S186 L207 S187 S188 S189 L208 L209 L210 L211 L212 S190 | S191 S192 L213 S193 S194 S195 L214 L215 L216 L217 L218 S196 | S197 S198 L219 S199 S200 S201 L220 L221 L222 L223 L224 S202 | S203 S204 L225 S205 S206 S207 S208 S209 S210 S211 L226 S212 S213 S214 S215 L227 S216 | L228 L229 L230 L231 L232 L233 | S217 S218 L234 S219 S220 S221 L235 L236 L237 L238 L239 S222 | S223 S224 L240 S225 S226 S227 L241 L242 L243 L244 L245 S228 | L246 L247 L248 L249 L250 L251 | L252 L253 L254 L255 L256 L257 | L258 L259 L260 L261 L262 L263 | L264 L265 L266 L267 L268 L269 L270 L271 L272 L273 | S229 L274 L275 L276 S230 S231 S232 S233 | S234 S235 S236 S237 | L277 L278 L279 L280 L281 L282 L283 L284 L285 L286 | S238 S239 L287 S240 S241 S242 S243 L288 L289 L290 S244 S245 S246 | S247 S248 L291 S249 S250 S251 L292 L293 L294 L295 L296 S252 | S253 S254 S255 S256 | S257 S258 S259 S260 | L297 L298 L299 L300 L301 S261 S262 S263 S264 L302 S265 S266 S267 S268 | L303 L304 L305 S269 S270 S271 L306 L307 L308 L309 L310 | S272 S273 L311 S274 S275 S276 S277 S278 S279 S280 S281 L312 S282 S283 S284 S285 S286 | L313 L314 L315 S287 S288 S289 S290 L316 L317 | S291 S292 L318 S293 S294 S295 S296 S297 S298 S299 L319 S300 S301 S302 S303 L320 S304 | S305 L321 L322 L323 S306 S307 S308 S309 | S310 S311 L324 S312 S313 S314 S315 S316 S317 S318 L325 S319 S320 S321 S322 L326 S323 | S324 S325 L327 S326 S327 S328 S329 S330 S331 S332 L328 S333 S334 S335 S336 L329 S337 | S338 S339 L330 S340 S341 S342 S343 S344 S345 S346 L331 S347 S348 S349 S350 L332 S351 | L333 L334 L335 L336 L337 L338 L339 L340 L341 L342 | L343 L344 L345 L346 L347 S352 S353 S354 S355 L348 S356 S357 S358 S359 | L349 L350 L351 L352 L353 L354 | L355 L356 L357 L358 L359 L360 L361 L362 L363 L364 | A17 L366 A18 L365 | A19 | A20 | A21 | A22 | A23 | A24 | A25 | A26 | A27 | A28 | A29 | A30 | A31 | A32 | A33 | A34 L368 A35 L367 | A36 L370 A37 L369 | L371 A38 L372 A39 L373 L374 L375 L376 L377 L378 L379 L380 L385 L386 L381 L382 | L381 A40 L380 L384 L383 | L386 L385 A40
sketch "Skizze7" plane through (0, 0, 0) normal (0, 1, 0) x (-1, 0, 0)
  line L0 (-15.9411, 18) -> (-15.9411, 0)
  line L1 (-26.1396, -3.9976) -> (-26, 0)
  line L2 (-15.9411, 0) -> (-23.4797, 0)
  line L3 (-15.9411, 0) -> (-8.4025, 0) construction
  line L4 (-23.4797, 0) -> (-22.1995, 11.4884)
  line L5 (-22.1995, 11.4884) -> (-15.9411, 18)
  point P0 (0, 0)
  dimension "d18" = 180
  constraints: 8 end point, 1 collinear, 1 horizontal
  measures "d18" angle of L2 L3
extrude "Extrusion6" cut sketch "Skizze7" along normal mid plane 23
sketch "Skizze8" plane through (22.1995, -11.5, 11.4884) normal (-0.9938, 0, -0.1107) x (-0.1107, 0, 0.9938)
  circle A0 centre (-7.3562, 11.5) radius 3.5
  point P0 (-8.9592, 11.5)
  dimension "d21" = 7
  constraints: 1 centre point
  measures "d21" diameter of A0
extrude "Extrusion7" cut sketch "Skizze8" against normal blind 23
